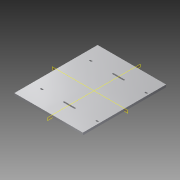
# Autodesk Inventor part: plate_base
Saved by Autodesk Inventor 2014 SP1 (Build 180222100, 222)
## iProperties
Created: 2016-09-05
Part Number: plate_base
Material: Aluminum 6061-AHC
Document SubType Name: Modeling
Designer: tguillod
Density: 2.71 g/cm^3
Appearance: Aluminum - Dark
Author: tguillod
Autodesk Inventor part; units mm, degrees
ref_plane "YZ Plane" through (0, 0, 0) normal (1, 0, 0) x (0, 1, 0)
ref_plane "XZ Plane" through (0, 0, 0) normal (0, 1, 0) x (-1, 0, 0)
ref_plane "XY Plane" through (0, 0, 0) normal (0, 0, 1) x (1, 0, 0)
sketch "Sketch1" plane through (0, 0, 0) normal (0, 0, 1) x (1, 0, 0)
  line L0 (0, 0) -> (146, 0)
  line L1 (146, 0) -> (146, 177.5)
  line L2 (146, 177.5) -> (0, 177.5)
  line L3 (0, 177.5) -> (0, 0)
  dimension "d0" = 146
  dimension "d1" = 177.5
  constraints: 8 end point, 2 parallel, 1 horizontal, 1 perpendicular
  measures "d0" distance of L1.end L2.end
  measures "d1" distance of L0.end L1.end
extrude "Extrusion1" add sketch "Sketch1" along normal blind 5
sketch "Sketch3" plane through (0, 0, 5) normal (0, 0, 1) x (1, 0, 0)
  line L0 (0, 0) -> (146, 0) projected
  line L1 (146, 0) -> (146, 177.5) projected
  line L2 (146, 177.5) -> (0, 177.5) projected
  line L3 (0, 177.5) -> (0, 0) projected
  line L4 (0, 141) -> (146, 141) construction
  line L5 (0, 36.5) -> (146, 36.5) construction
  line L6 (22, 177.5) -> (22, 0) construction
  line L7 (81, 0) -> (81, 177.5) construction
  line L8 (140, 177.5) -> (140, 0) construction
  line L9 (20.5, 142.5) -> (23.5, 142.5)
  line L10 (25, 141) -> (25, 141)
  line L11 (23.5, 139.5) -> (20.5, 139.5)
  line L12 (19, 141) -> (19, 141)
  line L13 (19, 142.5) -> (25, 139.5) construction
  line L14 (25, 142.5) -> (19, 139.5) construction
  line L15 (20.5, 38) -> (23.5, 38)
  line L16 (25, 36.5) -> (25, 36.5)
  line L17 (23.5, 35) -> (20.5, 35)
  line L18 (19, 36.5) -> (19, 36.5)
  line L19 (19, 38) -> (25, 35) construction
  line L20 (25, 38) -> (19, 35) construction
  line L21 (138.5, 142.5) -> (141.5, 142.5)
  line L22 (143, 141) -> (143, 141)
  line L23 (141.5, 139.5) -> (138.5, 139.5)
  line L24 (137, 141) -> (137, 141)
  line L25 (137, 142.5) -> (143, 139.5) construction
  line L26 (143, 142.5) -> (137, 139.5) construction
  line L27 (141.5, 38) -> (138.5, 38)
  line L28 (137, 36.5) -> (137, 36.5)
  line L29 (138.5, 35) -> (141.5, 35)
  line L30 (143, 36.5) -> (143, 36.5)
  line L31 (143, 38) -> (137, 35) construction
  line L32 (137, 38) -> (143, 35) construction
  arc A0 (20.5, 142.5) -> (19, 141) centre (20.5, 141) ccw
  arc A1 (25, 141) -> (23.5, 142.5) centre (23.5, 141) ccw
  arc A2 (23.5, 139.5) -> (25, 141) centre (23.5, 141) ccw
  arc A3 (19, 141) -> (20.5, 139.5) centre (20.5, 141) ccw
  arc A4 (20.5, 38) -> (19, 36.5) centre (20.5, 36.5) ccw
  arc A5 (25, 36.5) -> (23.5, 38) centre (23.5, 36.5) ccw
  arc A6 (23.5, 35) -> (25, 36.5) centre (23.5, 36.5) ccw
  arc A7 (19, 36.5) -> (20.5, 35) centre (20.5, 36.5) ccw
  arc A8 (141.5, 35) -> (143, 36.5) centre (141.5, 36.5) ccw
  arc A9 (137, 36.5) -> (138.5, 35) centre (138.5, 36.5) ccw
  arc A10 (138.5, 38) -> (137, 36.5) centre (138.5, 36.5) ccw
  arc A11 (143, 36.5) -> (141.5, 38) centre (141.5, 36.5) ccw
  arc A12 (138.5, 142.5) -> (137, 141) centre (138.5, 141) ccw
  arc A13 (137, 141) -> (138.5, 139.5) centre (138.5, 141) ccw
  arc A14 (143, 141) -> (141.5, 142.5) centre (141.5, 141) ccw
  arc A15 (141.5, 139.5) -> (143, 141) centre (141.5, 141) ccw
  line L33 (69.5, 142.5) -> (92.5, 142.5)
  line L34 (94, 141) -> (94, 141)
  line L35 (92.5, 139.5) -> (69.5, 139.5)
  line L36 (68, 141) -> (68, 141)
  line L37 (68, 142.5) -> (94, 139.5) construction
  line L38 (94, 142.5) -> (68, 139.5) construction
  line L39 (69.5, 38) -> (92.5, 38)
  line L40 (94, 36.5) -> (94, 36.5)
  line L41 (92.5, 35) -> (69.5, 35)
  line L42 (68, 36.5) -> (68, 36.5)
  line L43 (68, 38) -> (94, 35) construction
  line L44 (94, 38) -> (68, 35) construction
  arc A16 (69.5, 142.5) -> (68, 141) centre (69.5, 141) ccw
  arc A17 (68, 141) -> (69.5, 139.5) centre (69.5, 141) ccw
  arc A18 (92.5, 139.5) -> (94, 141) centre (92.5, 141) ccw
  arc A19 (94, 141) -> (92.5, 142.5) centre (92.5, 141) ccw
  arc A20 (69.5, 38) -> (68, 36.5) centre (69.5, 36.5) ccw
  arc A21 (68, 36.5) -> (69.5, 35) centre (69.5, 36.5) ccw
  arc A22 (92.5, 35) -> (94, 36.5) centre (92.5, 36.5) ccw
  arc A23 (94, 36.5) -> (92.5, 38) centre (92.5, 36.5) ccw
  point P0 (22, 141)
  point P1 (22, 36.5)
  point P2 (81, 36.5)
  point P3 (81, 141)
  point P4 (140, 141)
  point P5 (140, 36.5)
  dimension "d22" = 36.5
  dimension "d23" = 36.5
  dimension "d24" = 104.5
  dimension "d25" = 59
  dimension "d26" = 59
  dimension "d36" = 22
  dimension "d39" = 3
  dimension "d40" = 6
  dimension "d41" = 1.5
  dimension "d42" = 1.5
  dimension "d43" = 1.5
  dimension "d44" = 1.5
  dimension "d47" = 26
  dimension "d48" = 26
  dimension "d49" = 3
  dimension "d50" = 3
  dimension "d51" = 1.5
  dimension "d52" = 1.5
  constraints: 82 end point, 70 point on line, 48 point on circle, 48 tangent, 24 centre point, 18 equal radius, 13 parallel, 12 midpoint, 10 perpendicular, 6 equal length, 6 horizontal
  measures "d22" distance between parallel lines of L2 L4
  measures "d23" distance between parallel lines of L5 L0
  measures "d24" distance between parallel lines of L4 L5
  measures "d25" distance between parallel lines of L7 L6
  measures "d26" distance between parallel lines of L8 L7
  measures "d36" distance between parallel lines of L3 L6
  measures "d39" distance of L14.start L13.end
  measures "d40" distance of L13.start L14.start
  measures "d41" radius of A0
  measures "d42" radius of A4
  measures "d43" radius of A8
  measures "d44" radius of A12
  measures "d47" distance of L37.start L38.start
  measures "d48" distance of L43.start L44.start
  measures "d49" distance of L38.start L37.end
  measures "d50" distance of L44.start L43.end
  measures "d51" radius of A16
  measures "d52" radius of A20
extrude "Extrusion4" cut sketch "Sketch3" against normal blind 10 contours L9 A1 A2 L11 A3 A0 | L15 A5 A6 L17 A7 A4 | L21 A14 A15 L23 A13 A12 | A11 A8 L29 A9 A10 L27 | L33 A19 A18 L35 A17 A16 | L39 A23 A22 L41 A21 A20
ref_plane "Work Plane1" through (81, 38, 5) normal (1, 0, 0) x (0, 0, -1)
ref_plane "Work Plane2" through (69.5, 88.75, 5) normal (0, -1, 0) x (1, 0, 0)
body "Solid1"
